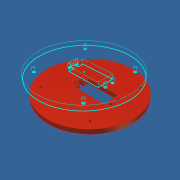
# Autodesk Inventor part: Acrylic_rotationServoMount
Saved by Autodesk Inventor 2012 (Build 160160000, 160)
## iProperties
Created: 2014-03-29
Part Number: Acrylic_rotationServoMount
Material: Default
Document SubType Name: Modeling
Designer: Admin
Density: 1 g/cm^3
Author: Admin
Autodesk Inventor part; units mm, degrees
ref_plane "YZ Plane" through (0, 0, 0) normal (1, 0, 0) x (0, 1, 0)
ref_plane "XZ Plane" through (0, 0, 0) normal (0, 1, 0) x (-1, 0, 0)
ref_plane "XY Plane" through (0, 0, 0) normal (0, 0, 1) x (1, 0, 0)
sketch "Sketch1" plane through (0, 0, 0) normal (0, 0, 1) x (1, 0, 0)
  circle A0 centre (0, 0) radius 60
  dimension "d0" = 120
  constraints: 1 centre point, 1 coincident
  measures "d0" diameter of A0
extrude "Extrusion1" add sketch "Sketch1" along normal blind 5.8
sketch "Sketch2" plane through (0, 0, 5.8) normal (0, 0, 1) x (1, 0, 0)
  circle A0 centre (0, 0) radius 60 projected
  circle A1 centre (0, 0) radius 6.4031
  constraints: 1 centre point, 1 coincident
extrude "Extrusion2" cut sketch "Sketch2" against normal through all contours A1
sketch "Sketch3" plane through (0, 0, 0) normal (0, 0, -1) x (-1, 0, 0)
  circle A0 centre (0, 0) radius 6.4031 projected
  circle A1 centre (0, 0) radius 3
  line L0 (12.25, 9.9) -> (-28.05, 9.9)
  line L1 (-28.05, -9.9) -> (12.25, -9.9)
  line L2 (-28.05, 9.9) -> (-28.05, -9.9)
  line L3 (18.25, 2.5) -> (12.25, 2.5)
  line L4 (18.25, -2.5) -> (18.25, 2.5)
  line L5 (12.25, -2.5) -> (18.25, -2.5)
  line L6 (12.25, 2.5) -> (12.25, 9.9)
  line L7 (12.25, -9.9) -> (12.25, -2.5)
  constraints: 16 end point, 4 horizontal, 4 vertical, 1 centre point, 10 other
extrude "Extrusion3" cut sketch "Sketch3" against normal through all contours L6 L3 L4 L5 L7 L1 L2 L0
sketch "Sketch4" plane through (0, 0, 5.8) normal (0, 0, 1) x (1, 0, 0)
  circle A0 centre (-16.6, 5) radius 2.5
  circle A1 centre (-16.6, -5) radius 2.5
  circle A2 centre (32.4, -5) radius 2.5
  circle A3 centre (32.4, 5) radius 2.5
  circle A4 centre (-16.6, 5) radius 1.5
  circle A5 centre (-16.6, -5) radius 1.5
  circle A6 centre (32.4, 5) radius 1.5
  circle A7 centre (32.4, -5) radius 1.5
  dimension "d7" = 3
  dimension "d8" = 3
  dimension "d9" = 3
  dimension "d10" = 3
  constraints: 8 centre point, 4 coincident, 8 other
  measures "d7" diameter of A4
  measures "d8" diameter of A5
  measures "d9" diameter of A6
  measures "d10" diameter of A7
extrude "Extrusion4" cut sketch "Sketch4" against normal through all contours A4 | A5 | A6 | A7
sketch "Sketch5" plane through (0, 0, 5.8) normal (0, 0, 1) x (1, 0, 0)
  circle A0 centre (0, 0) radius 60 projected
  circle A1 centre (-35.355, 35.355) radius 1.5
  line L0 (0, -84) -> (0, 84) projected
  line L1 (-84, 0) -> (84, 0) projected
  circle A2 centre (-35.355, -35.355) radius 1.5
  circle A3 centre (35.355, -35.355) radius 1.5
  circle A4 centre (35.355, 35.355) radius 1.5
  dimension "d13" = 3
  dimension "d15" = 35.355
  dimension "d17" = 35.355
  dimension "d20" = 360
  constraints: 4 centre point, 9 other
  measures "d13" diameter of A1
  measures "d15" distance from line of L0 A1.centre
  measures "d17" distance from line of L1 A1.centre
extrude "Extrusion5" cut sketch "Sketch5" against normal through all contours A1 | A2 | A3 | A4
sketch "Sketch6" plane through (0, 0, 0) normal (0, 0, -1) x (-1, 0, 0)
  circle A0 centre (-35.355, 35.355) radius 1.5 projected
  circle A1 centre (-35.355, -35.355) radius 1.5 projected
  circle A2 centre (35.355, -35.355) radius 1.5 projected
  circle A3 centre (35.355, 35.355) radius 1.5 projected
  circle A4 centre (-32.4, 5) radius 1.5 projected
  circle A5 centre (16.6, -5) radius 1.5 projected
  circle A6 centre (16.6, 5) radius 1.5 projected
  circle A7 centre (-32.4, -5) radius 1.5 projected
  line L0 (-28.05, -9.9) -> (-28.05, 9.9) projected
  line L1 (-28.05, 9.9) -> (12.25, 9.9) projected
  line L2 (12.25, 9.9) -> (12.25, 2.5) projected
  line L3 (12.25, 2.5) -> (18.25, 2.5) projected
  line L4 (18.25, 2.5) -> (18.25, -2.5) projected
  line L5 (18.25, -2.5) -> (12.25, -2.5) projected
  line L6 (12.25, -2.5) -> (12.25, -9.9) projected
  line L7 (12.25, -9.9) -> (-28.05, -9.9) projected
  circle A8 centre (0, 0) radius 60 projected
  circle A9 centre (35.355, 35.355) radius 1.385
  circle A10 centre (-35.355, 35.355) radius 1.5 projected
  circle A11 centre (-35.355, -35.355) radius 1.5 projected
  circle A12 centre (35.355, -35.355) radius 1.5 projected
  circle A13 centre (35.355, 35.355) radius 1.5 projected
  circle A14 centre (-32.4, 5) radius 1.5 projected
  circle A15 centre (16.6, -5) radius 1.5 projected
  circle A16 centre (16.6, 5) radius 1.5 projected
  circle A17 centre (-32.4, -5) radius 1.5 projected
  line L8 (-28.05, -9.9) -> (-28.05, 9.9) projected
  line L9 (-28.05, 9.9) -> (12.25, 9.9) projected
  line L10 (12.25, 9.9) -> (12.25, 2.5) projected
  line L11 (12.25, 2.5) -> (18.25, 2.5) projected
  line L12 (18.25, 2.5) -> (18.25, -2.5) projected
  line L13 (18.25, -2.5) -> (12.25, -2.5) projected
  line L14 (12.25, -2.5) -> (12.25, -9.9) projected
  line L15 (12.25, -9.9) -> (-28.05, -9.9) projected
  circle A18 centre (0, 0) radius 60 projected
  line L16 (-28.05, 9.9) -> (-28.05, -9.9) projected
  line L17 (-28.05, -9.9) -> (-28.05, 9.9) projected
  line L18 (12.25, 9.9) -> (-28.05, 9.9) projected
  line L19 (-28.05, 9.9) -> (12.25, 9.9) projected
  circle A19 centre (-32.4, -5) radius 1.5 projected
  circle A20 centre (-32.4, -5) radius 1.5 projected
  circle A21 centre (35.355, -35.355) radius 1.385
  circle A22 centre (-35.355, 35.355) radius 1.385
  circle A23 centre (-35.355, -35.355) radius 1.385
  constraints: 4 centre point, 8 other
equation "\"d17\" = d15"
body "Solid1"
